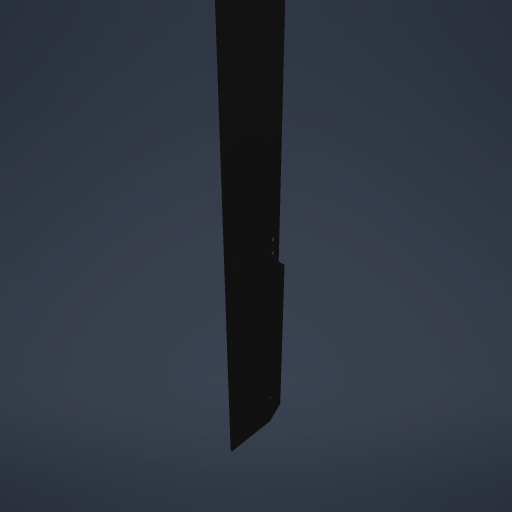
# Autodesk Inventor part: Side Guard
Saved by Autodesk Inventor 2023 (Build 270158000, 158)
## iProperties
Created: 2022-10-29
Part Number: Side Guard
Material: Generic
Document SubType Name: Modeling
Designer: alex
Density: 1 g/cm^3
Appearance: Default
Author: alex
Autodesk Inventor part; units mm, degrees
ref_plane "YZ Plane" through (0, 0, 0) normal (1, 0, 0) x (0, 1, 0)
ref_plane "XZ Plane" through (0, 0, 0) normal (0, 1, 0) x (-1, 0, 0)
ref_plane "XY Plane" through (0, 0, 0) normal (0, 0, 1) x (1, 0, 0)
sketch "Sketch1" plane through (0, 0, 0) normal (1, 0, 0) x (0, 1, 0)
  line L0 (22.9119, 0) -> (-383.4881, 0)
  line L1 (-383.4881, 0) -> (-383.4881, 57.15)
  line L2 (-383.4881, 57.15) -> (22.9119, 57.15)
  line L3 (22.9119, 57.15) -> (22.9119, 0)
  line L4 (22.9119, 0) -> (22.9119, 1.6002)
  line L5 (-383.4881, 22.987) -> (-383.4881, 2.413)
  line L6 (22.2741, 57.15) -> (-5.0281, 57.15)
  circle A0 centre (16.5619, 6.35) radius 2.1463
  circle A1 centre (-351.7381, 6.35) radius 2.1463
  circle A2 centre (-173.8111, 6.35) radius 2.1463
  circle A3 centre (-186.6381, 6.35) radius 2.1463
  circle A4 centre (19.8639, 49.53) radius 1.27
  circle A5 centre (13.2599, 49.53) radius 1.27
  circle A6 centre (-176.4781, 44.7802) radius 1.27
  circle A7 centre (-182.4471, 44.7802) radius 1.27
  circle A8 centre (-380.4401, 49.53) radius 1.27
  circle A9 centre (-373.8361, 49.53) radius 1.27
  line L7 (-383.4881, 0) -> (-370.7881, 0) construction
  line L8 (22.9119, 6.35) -> (16.5619, 0)
  line L9 (-383.4881, 6.35) -> (-370.0177, -7.1204)
  line L10 (-383.4881, 6.35) -> (-364.4381, 6.35) construction
  line L11 (-370.0177, -7.1204) -> (-204.9177, -7.1204)
  line L12 (-204.9177, -7.1204) -> (-197.7973, 0)
  point P0 (0, 0)
  point P1 (-187.7276, 0)
  dimension "d0" = 4.2926
  dimension "d1" = 6.35
  dimension "d2" = 6.35
  dimension "d3" = 4.2926
  dimension "d4" = 31.75
  dimension "d5" = 6.35
  dimension "d6" = 4.2926
  dimension "d7" = 6.35
  dimension "d8" = 4.2926
  dimension "d9" = 6.35
  dimension "d10" = 196.723
  dimension "d11" = 196.85
  dimension "d12" = 2.54
  dimension "d13" = 3.048
  dimension "d14" = 7.62
  dimension "d15" = 2.54
  dimension "d16" = 7.62
  dimension "d17" = 9.652
  dimension "d18" = 2.54
  dimension "d19" = 12.3698
  dimension "d20" = 199.39
  dimension "d21" = 2.54
  dimension "d22" = 12.3698
  dimension "d23" = 5.969
  dimension "d24" = 2.54
  dimension "d25" = 7.62
  dimension "d26" = 3.048
  dimension "d27" = 2.54
  dimension "d28" = 7.62
  dimension "d29" = 9.652
  dimension "d36" = 19.05
  dimension "d37" = 45
  dimension "d38" = 165.1
  dimension "d39" = 135
  constraints: 26 end point, 10 centre point, 5 point on line, 3 collinear, 3 horizontal, 3 parallel, 1 equal length, 1 perpendicular
  measures "d0" diameter of A0
  measures "d1" distance from line of L0 A0.centre
  measures "d2" distance from line of L3 A0.centre
  measures "d3" diameter of A1
  measures "d4" distance from line of L1 A1.centre
  measures "d5" distance from line of L0 A1.centre
  measures "d6" diameter of A2
  measures "d7" distance from line of L0 A2.centre
  measures "d8" diameter of A3
  measures "d9" distance from line of L0 A3.centre
  measures "d10" distance from line of L3 A2.centre
  measures "d11" distance from line of L1 A3.centre
  measures "d12" diameter of A4
  measures "d13" distance from line of L3 A4.centre
  measures "d14" distance from line of L2 A4.centre
  measures "d15" diameter of A5
  measures "d16" distance from line of L6 A5.centre
  measures "d17" distance from line of L3 A5.centre
  measures "d18" diameter of A6
  measures "d19" distance from line of A6.centre L2
  measures "d20" distance from line of L3 A6.centre
  measures "d21" diameter of A7
  measures "d22" distance from line of L2 A7.centre
  measures "d23" distance of A7.centre A6.centre
  measures "d24" diameter of A8
  measures "d25" distance from line of L2 A8.centre
  measures "d26" distance from line of L1 A8.centre
  measures "d27" diameter of A9
  measures "d28" distance from line of L2 A9.centre
  measures "d29" distance from line of L1 A9.centre
  measures "d36" distance of L9.start L9.end
  measures "d37" angle of L9 L10
  measures "d38" distance of L9.end L11.end
  measures "d39" angle of L11 L9
extrude "Extrusion1" add sketch "Sketch1" along normal blind 1.5875 contours L0 L9 L1 L2 L3 L8 | L12 L11 L9 L0
body "Solid1"
